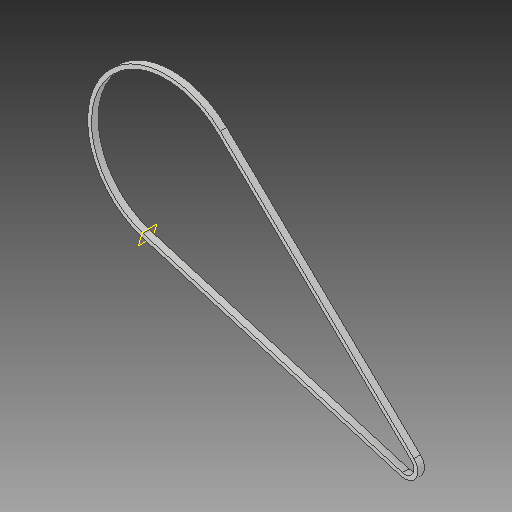
# Autodesk Inventor part: Cadena2
Saved by Autodesk Inventor 2019.2 (Build 232265000, 265)
## iProperties
Created: 2017-12-04
Part Number: Cadena2
Material: Generic
Document SubType Name: Modeling
Designer: eroldan
Density: 1 g/cm^3
Appearance: Default
Author: eroldan
Autodesk Inventor part; units mm, degrees
ref_plane "YZ Plane" through (0, 0, 0) normal (1, 0, 0) x (0, 1, 0)
ref_plane "XZ Plane" through (0, 0, 0) normal (0, 1, 0) x (-1, 0, 0)
ref_plane "Work Plane6" through (-3.713488, 14.864291, 104.198762) normal (0, 0, 1) x (0.9994468, -0.0332592, 0)
sketch "Sketch1" plane through (-3.713488, 14.864291, 104.198762) normal (0, 0, 1) x (0.9994468, -0.0332592, 0)
  arc A0 (131.880776, 188.685572) -> (21.678185, -9.803405) centre (53.87003, 102.160585) ccw
  line L0 (131.880776, 188.685572) -> (436.873817, -86.295513)
  circle A1 centre (53.87003, 102.160585) radius 17.5
  arc A2 (21.678185, -9.803405) -> (24.529382, -10.584155) centre (53.87003, 102.160585) ccw
  arc A3 (421.49686, -114.765827) -> (436.873817, -86.295513) centre (425.724642, -98.66153) ccw
  line L1 (21.678185, -9.803405) -> (421.49686, -114.765827)
  constraints: 6 point on circle, 4 centre point, 4 end point, 3 tangent, 1 coincident, 8 other
ref_plane "Work Plane13" through (20.450302, 3.470164, 104.198762) normal (0.9582447, -0.2859495, 0) x (0.2859495, 0.9582447, 0)
sketch "Sketch2" plane through (82.301795, 210.740594, 104.198762) normal (0.9582447, -0.2859495, 0) x (0.2859495, 0.9582447, 0)
  line L0 (-213.329407, -5) -> (-219.329407, -5)
  line L1 (-219.329407, -5) -> (-219.329407, 5)
  line L2 (-219.329407, 5) -> (-213.329407, 5)
  line L3 (-213.329407, 5) -> (-213.329407, -5)
  line L4 (-219.329407, -5) -> (-213.329407, 5) construction
  line L5 (-219.329407, 5) -> (-213.329407, -5) construction
  point P0 (-216.329407, 0)
  point P1 (-216.329407, 0)
  point P2 (-216.329407, 0)
  point P3 (-216.329407, 0)
  dimension "d0" = 6
  dimension "d1" = 10
  constraints: 12 end point, 2 parallel, 1 coincident, 1 horizontal, 1 midpoint, 1 perpendicular
  measures "d0" distance of L1.end L2.end
  measures "d1" distance of L0.end L1.end
sweep "Sweep1" add profiles "Sketch2" path "Sketch1" path curves L1 A3 L0 A0
body "Solid1"
